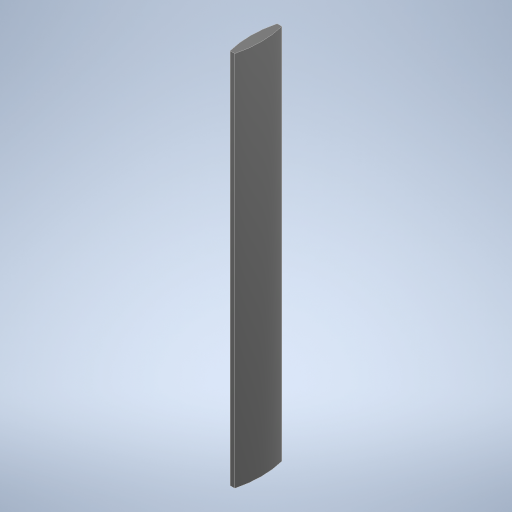
# Autodesk Inventor part: Antenna
Saved by Autodesk Inventor 2024.2 (Build 282272000, 272)
## iProperties
Created: 2024-01-25
Part Number: Antenna
Material: Acetal Resin, Black
Document SubType Name: Modeling
Designer: airso
Density: 1.425 g/cm^3
Appearance: Smooth - Black
Author: airso
Autodesk Inventor part; units mm, degrees
ref_plane "YZ Plane" through (0, 0, 0) normal (1, 0, 0) x (0, 1, 0)
ref_plane "XZ Plane" through (0, 0, 0) normal (0, 1, 0) x (-1, 0, 0)
ref_plane "XY Plane" through (0, 0, 0) normal (0, 0, 1) x (1, 0, 0)
sketch "Sketch1" plane through (0, 0, 0) normal (0, 1, 0) x (-1, 0, 0)
  arc A0 (0, -12.7) -> (0, 0) centre (-24.5934, -6.35) ccw
  line L0 (0, 0) -> (-1.27, 0)
  line L1 (0, -12.7) -> (-1.27, -12.7)
  arc A1 (-1.27, 0) -> (-1.27, -12.7) centre (23.3234, -6.35) ccw
  dimension "d0" = 12.7
  dimension "d1" = 25.4
  dimension "d2" = 1.27
  dimension "d3" = 25.4
  constraints: 4 end point, 4 point on circle, 2 centre point, 2 horizontal
  measures "d0" distance of L0.start L1.start
  measures "d1" radius of A0
  measures "d2" distance of L0.start L0.end
  measures "d3" radius of A1
extrude "Extrusion1" add sketch "Sketch1" along normal blind 101.6
body "Solid1"
